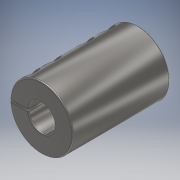
# Autodesk Inventor part: MCLX-12-12-F
Saved by Autodesk Inventor 2018 (Build 220112000, 112)
## iProperties
Created: 2018-04-10
Part Number: MCLX-12-12-F
Material: Steel, Carbon
Document SubType Name: Modeling
Designer: P136265
Density: 7.85 g/cm^3
Appearance: Semi-Polished
Author: P136265
Autodesk Inventor part; units mm, degrees
ref_plane "YZ Plane" through (0, 0, 0) normal (1, 0, 0) x (0, 1, 0)
ref_plane "XZ Plane" through (0, 0, 0) normal (0, 1, 0) x (-1, 0, 0)
sketch "Sketch1" plane through (0, 0, 0) normal (0, 1, 0) x (-1, 0, 0)
  arc A0 (14.4914, 0.5) -> (14.4914, -0.5) centre (0, 0) ccw
  arc A1 (6.0042, 0.5) -> (6.0042, -0.5) centre (0, 0) ccw
  line L0 (6.0042, 0.5) -> (14.4914, 0.5)
  line L1 (6.0042, -0.5) -> (14.4914, -0.5)
  dimension "d0" = 29
  dimension "d1" = 12.05
  dimension "d3" = 1
  dimension "d4" = 0.5
  constraints: 4 coincident, 4 end point, 4 point on circle, 2 centre point, 2 horizontal
  measures "d0" diameter of A0
  measures "d1" diameter of A1
  measures "d3" distance between parallel lines of L1 L0
  measures "d4" distance from line of point (0, 0) L0
extrude "Extrusion1" add sketch "Sketch1" along normal mid plane 45
ref_plane "Work Plane1" through (0, 0, 4) normal (0, 0, 1) x (1, 0, 0)
sketch "Sketch4" plane through (0, 0, 4) normal (0, 0, 1) x (1, 0, 0)
  line L0 (0, 0) -> (0, 40) construction
  line L1 (-14.4914, -22.5) -> (14.5, -22.5) construction
  line L2 (14.5, 22.5) -> (-14.4914, 22.5) construction
  circle A0 centre (-10.6, 17.5) radius 3.5
  circle A1 centre (-10.6, -17.5) radius 3.5
  line L3 (-10.6, 17.5) -> (-10.6, -17.5) construction
  circle A2 centre (-10.6, -7.5) radius 3.5
  circle A3 centre (-10.6, 7.5) radius 3.5
  dimension "d24" = 40
  dimension "d25" = 7
  dimension "d26" = 5
  dimension "d28" = 7
  dimension "d29" = 5
  dimension "d30" = 7
  dimension "d31" = 7
  dimension "d32" = 10
  dimension "d33" = 10
  dimension "d34" = 10.6
  constraints: 4 centre point, 4 end point, 2 point on line, 2 vertical
  measures "d24" distance of L0.start L0.end
  measures "d25" diameter of A0
  measures "d26" distance from line of L2 L3.start
  measures "d28" diameter of A1
  measures "d29" distance from line of L1 L3.end
  measures "d30" diameter of A2
  measures "d31" diameter of A3
  measures "d32" distance of L3.end A2.centre
  measures "d33" distance of L3.start A3.centre
  measures "d34" distance between parallel lines of L0 L3
extrude "Extrusion3" cut sketch "Sketch4" along normal blind 45
mirror "Mirror1" about plane through (0, 0, 0) normal (0, 0, 1) of "Extrusion3"
sketch "Sketch5" plane through (0, 0, 4) normal (0, 0, 1) x (1, 0, 0)
  arc A0 (-13.9374, 6.4455) -> (-13.9374, 8.5545) centre (-10.6, 7.5) ccw construction
  arc A1 (-13.9374, -8.5545) -> (-13.9374, -6.4455) centre (-10.6, -7.5) ccw construction
  arc A2 (-13.9374, -18.5545) -> (-13.9374, -16.4455) centre (-10.6, -17.5) ccw construction
  arc A3 (-13.9374, 16.4455) -> (-13.9374, 18.5545) centre (-10.6, 17.5) ccw construction
  point P0 (0, 0)
  constraints: 1 vertical alignment
hole "Hole1" at (-10.6, 17.5, 4) at (-10.6, 7.5, 4) at (-10.6, -7.5, 4) at (-10.6, -17.5, 4) direction (0, 0, -1) diameter 4 end through all
fillet "Fillet1" radius 0.5 4 edges at (14.5, 22.5, 0) (14.5, -22.5, 0) (6.025, 22.5, 0) (6.025, -22.5, 0)
body "Solid1"
